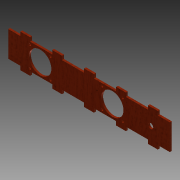
# Autodesk Inventor part: Panel4_FanCutout
Saved by Autodesk Inventor 2015 (Build 190159000, 159)
## iProperties
Created: 2014-08-06
Part Number: Panel4_FanCutout
Material: Wood (Oak)
Document SubType Name: Modeling
Designer: Patrick Camilleri
Density: 0.76 g/cm^3
Appearance: White Oak - Natural Medium Gloss
Author: Patrick Camilleri
Autodesk Inventor part; units mm, degrees
ref_plane "YZ Plane" through (0, 0, 0) normal (1, 0, 0) x (0, 1, 0)
ref_plane "XZ Plane" through (0, 0, 0) normal (0, 1, 0) x (-1, 0, 0)
ref_plane "XY Plane" through (0, 0, 0) normal (0, 0, 1) x (1, 0, 0)
sketch "Sketch1" plane through (0, 0, 0) normal (0, 1, 0) x (-1, 0, 0)
  line L0 (20.15, 126.45) -> (-20.15, 126.45)
  line L1 (-20.15, 126.45) -> (-20.15, -126.45)
  line L2 (-20.15, -126.45) -> (20.15, -126.45)
  line L3 (20.15, -126.45) -> (20.15, 126.45)
  line L4 (20.15, 126.45) -> (-20.15, -126.45) construction
  line L5 (-20.15, 126.45) -> (20.15, -126.45) construction
  point P0 (0, 0)
  point P1 (0, 0)
  dimension "d0" = 40.3
  dimension "d1" = 252.9
  constraints: 12 end point, 3 midpoint, 2 parallel, 1 horizontal, 1 perpendicular
  measures "d0" distance of L2.end L1.end
  measures "d1" distance of L1.end L0.end
extrude "Extrusion1" add sketch "Sketch1" along normal blind 3
sketch "Sketch3" plane through (0, 0, 0) normal (0, -1, 0) x (1, 0, 0)
  line L0 (-20.15, 126.45) -> (20.15, 126.45) projected
  line L1 (-16.15, 52.45) -> (15.85, 52.45) construction
  line L2 (15.85, 52.45) -> (15.85, 20.45) construction
  line L3 (15.85, 20.45) -> (-16.15, 20.45) construction
  line L4 (-16.15, 20.45) -> (-16.15, 52.45) construction
  line L5 (-16.15, 52.45) -> (15.85, 20.45) construction
  line L6 (15.85, 52.45) -> (-16.15, 20.45) construction
  line L7 (20.15, -126.45) -> (-20.15, -126.45) projected
  line L8 (16.15, -92.45) -> (-15.85, -92.45) construction
  line L9 (-15.85, -92.45) -> (-15.85, -60.45) construction
  line L10 (-15.85, -60.45) -> (16.15, -60.45) construction
  line L11 (16.15, -60.45) -> (16.15, -92.45) construction
  line L12 (16.15, -92.45) -> (-15.85, -60.45) construction
  line L13 (-15.85, -92.45) -> (16.15, -60.45) construction
  point P0 (0, 0)
  point P1 (-0.15, 36.45)
  point P2 (0.15, -76.45)
  dimension "d69" = 32
  dimension "d70" = 32
  dimension "d71" = 90
  dimension "d102" = 32
  dimension "d103" = 32
  dimension "d104" = 50
  constraints: 24 end point, 4 midpoint, 4 parallel, 2 coincident, 2 horizontal, 2 perpendicular
  measures "d69" distance of L2.end L3.end
  measures "d70" distance of L1.end L2.end
  measures "d71" distance from line of point (-0.15, 36.45) L0
  measures "d102" distance of L9.end L10.end
  measures "d103" distance of L8.end L9.end
  measures "d104" distance from line of point (0.15, -76.45) L7
hole "Hole2" at (15.85, 0, 52.45) at (16.15, 0, -60.45) direction (0, 1, 0) diameter 3.5 end through all
pattern_linear "Rectangular Pattern1" count 2 spacing 32 along (-1, 0, 0) count 2 spacing 32 along (0, 0, -1) of "Hole2"
sketch "Sketch5" plane through (0, 0, 0) normal (0, -1, 0) x (1, 0, 0)
  circle A0 centre (15.85, 20.45) radius 1.75 projected
  circle A1 centre (-16.15, 52.45) radius 1.75 projected
  line L0 (-16.15, 52.45) -> (15.85, 20.45) construction
  circle A2 centre (-0.15, 36.45) radius 17.5
  circle A3 centre (16.15, -92.45) radius 1.75 projected
  circle A4 centre (-15.85, -60.45) radius 1.75 projected
  line L1 (-15.85, -60.45) -> (16.15, -92.45) construction
  circle A5 centre (0.15, -76.45) radius 17.5
  line L2 (-20.15, 126.45) -> (20.15, 126.45) projected
  circle A6 centre (-0.15, 96.45) radius 4
  point P0 (0, 0)
  dimension "d86" = 35
  dimension "d105" = 35
  dimension "d106" = 8
  dimension "d107" = 30
  constraints: 4 end point, 3 centre point, 2 midpoint
  measures "d86" diameter of A2
  measures "d105" diameter of A5
  measures "d106" diameter of A6
  measures "d107" distance from line of A6.centre L2
extrude "Extrusion4" cut sketch "Sketch5" against normal through all contours A2 | A5 | A6
sketch "Sketch6" plane through (0, 0, 0) normal (0, -1, 0) x (1, 0, 0)
  line L0 (-20.15, -126.45) -> (-20.15, 126.45) projected
  line L1 (20.15, 126.45) -> (20.15, -126.45) projected
  line L2 (26.15, 7.65) -> (20.15, 7.65)
  line L3 (20.15, 7.65) -> (20.15, -7.65)
  line L4 (20.15, -7.65) -> (26.15, -7.65)
  line L5 (26.15, -7.65) -> (26.15, 7.65)
  line L6 (26.15, 7.65) -> (20.15, -7.65) construction
  line L7 (20.15, 7.65) -> (26.15, -7.65) construction
  line L8 (-20.15, 7.65) -> (-26.15, 7.65)
  line L9 (-26.15, 7.65) -> (-26.15, -7.65)
  line L10 (-26.15, -7.65) -> (-20.15, -7.65)
  line L11 (-20.15, -7.65) -> (-20.15, 7.65)
  line L12 (-20.15, 7.65) -> (-26.15, -7.65) construction
  line L13 (-26.15, 7.65) -> (-20.15, -7.65) construction
  point P0 (0, 0)
  point P1 (23.15, 0)
  point P2 (-20.15, 0)
  point P3 (20.15, 0)
  dimension "d90" = 6
  dimension "d91" = 15.3
  dimension "d92" = 6
  dimension "d93" = 15.3
  constraints: 24 end point, 6 midpoint, 4 parallel, 2 horizontal, 2 perpendicular
  measures "d90" distance of L4.end L3.end
  measures "d91" distance of L3.end L2.end
  measures "d92" distance of L10.end L9.end
  measures "d93" distance of L9.end L8.end
extrude "Extrusion5" add sketch "Sketch6" against normal blind 3
pattern_linear "Rectangular Pattern2" count 3 spacing 50 along (0, 0, 1) of "Extrusion5"
pattern_linear "Rectangular Pattern3" count 3 spacing 50 along (0, 0, -1) of "Extrusion5"
equation "\"kerf\" = 0.15"
body "Solid1"
